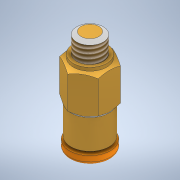
# Autodesk Inventor part: SMC10-32UNF-1-8 KQ2H01-32N RS 840-4665
Saved by Autodesk Inventor 2021 (Build 250183000, 183)
## iProperties
Created: 2020-07-29
Part Number: SMC10-32UNF-1-8 KQ2H01-32N RS 840-4665
Material: Generic
Document SubType Name: Modeling
Designer: jgray
Density: 1 g/cm^3
Appearance: Default
Author: jgray
Autodesk Inventor part; units mm, degrees
ref_plane "YZ Plane" through (0, 0, 0) normal (1, 0, 0) x (0, 1, 0)
ref_plane "XZ Plane" through (0, 0, 0) normal (0, 1, 0) x (-1, 0, 0)
ref_plane "XY Plane" through (0, 0, 0) normal (0, 0, 1) x (1, 0, 0)
sketch "Sketch1" plane through (0, 0, 0) normal (0, 1, 0) x (-1, 0, 0)
  circle A0 centre (0, 0) radius 4.041452
  line L0 (4.041452, 0) -> (2.020726, -3.5)
  line L1 (2.020726, -3.5) -> (-2.020726, -3.5)
  line L2 (-2.020726, -3.5) -> (-4.041452, 0)
  line L3 (-4.041452, 0) -> (-2.020726, 3.5)
  line L4 (-2.020726, 3.5) -> (2.020726, 3.5)
  line L5 (2.020726, 3.5) -> (4.041452, 0)
  dimension "d0" = 7
  constraints: 12 end point, 2 coincident, 1 horizontal alignment, 15 other
  measures "d0" distance between parallel lines of L3 L0
extrude "Extrusion1" add sketch "Sketch1" along normal blind 7
chamfer "Chamfer1" distance 1 angle 30 1 edges at (4.0415, 7, 0) measured on face at (3.5415, 7, 0)
chamfer "Chamfer2" distance 1 angle 30 1 edges at (4.0415, 0, 0) measured on face at (3.5415, 0, 0)
sketch "Sketch2" plane through (0, 0, 0) normal (0, -1, 0) x (1, 0, 0)
  circle A0 centre (0, 0) radius 4.041452
  circle A1 centre (0, 0) radius 4.041452
  line L0 (0, 4.041452) -> (3.5, 2.020726)
  line L1 (3.5, 2.020726) -> (3.5, -2.020726)
  line L2 (3.5, -2.020726) -> (0, -4.041452)
  line L3 (0, -4.041452) -> (-3.5, -2.020726)
  line L4 (-3.5, -2.020726) -> (-3.5, 2.020726)
  line L5 (-3.5, 2.020726) -> (0, 4.041452)
  point P0 (-3.5, 2.020726)
  point P1 (-3.5, 2.020726)
  point P2 (0, -4.041452)
  point P3 (0, -4.041452)
  constraints: 12 end point, 1 coincident, 1 vertical alignment, 14 other
extrude "Extrusion2" cut sketch "Sketch2" against normal blind 7 contours A0 L1 | L0 A0 | A0 L2 | L5 A0 | A0 L3 | L4 A0
sketch "Sketch3" plane through (0, 0, 0) normal (0, -1, 0) x (1, 0, 0)
  circle A0 centre (0, 0) radius 3.45
  dimension "d11" = 6.9
  constraints: 1 centre point, 1 coincident
  measures "d11" diameter of A0
extrude "Extrusion3" add sketch "Sketch3" along normal blind 5.3
fillet "Fillet1" radius 0.5 1 edges at (3.0415, 0, 0)
sketch "Sketch4" plane through (0, -5.3, 0) normal (0, -1, 0) x (1, 0, 0)
  circle A0 centre (0, 0) radius 2.25
  dimension "d15" = 4.5
  constraints: 1 centre point, 1 coincident
  measures "d15" diameter of A0
extrude "Extrusion4" add sketch "Sketch4" along normal blind 0.5
sketch "Sketch5" plane through (0, -5.8, 0) normal (0, -1, 0) x (1, 0, 0)
  circle A0 centre (0, 0) radius 2.25 projected
  circle A1 centre (0, 0) radius 3.7
  dimension "d18" = 7.4
  constraints: 1 centre point, 1 coincident
  measures "d18" diameter of A1
extrude "Extrusion5" add sketch "Sketch5" along normal blind 1.5 contours A0 | A1
fillet "Fillet2" radius 0.5 1 edges at (-3.7, -7.3, 0)
sketch "Sketch6" plane through (0, 7, 0) normal (0, 1, 0) x (1, 0, 0)
  circle A0 centre (0, 0) radius 3.041452
  constraints: 1 centre point, 1 coincident
extrude "Extrusion6" add sketch "Sketch6" along normal blind 0.6
sketch "Sketch7" plane through (0, 7.6, 0) normal (0, 1, 0) x (1, 0, 0)
  circle A0 centre (0, 0) radius 2.413
  dimension "d24" = 4.826
  constraints: 1 centre point, 1 coincident
  measures "d24" diameter of A0
extrude "Extrusion7" add sketch "Sketch7" along normal blind 3.5
thread "Thread1" size "10-32 UNF" class "2A" standard "ANSI Unified Screw Threads" length 15.103
chamfer "Chamfer3" distance 0.8 angle 30 1 edges at (-2.413, 11.1, 0) measured on face at (-1.913, 11.1, 0)
body "Solid1"
